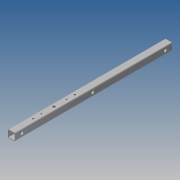
# Autodesk Inventor part: 2f2al
Saved by Autodesk Inventor 2014 SP1 (Build 180222100, 222)
## iProperties
Company: HERA Project
Created: 2013-06-27
Part Number: 2f2al
Material: Steel
Description: Feed backplane support crosspiece
Document SubType Name: Modeling
Designer: David DeBoer
Mass: 345.097 g
Surface Area: 540.887 cm^2
Volume: 43.9614 cm^3
Density: 7.85 g/cm^3
Appearance: Steel
Title: Feed backplane cross
Author: David DeBoer
Autodesk Inventor part; units mm, degrees
ref_plane "YZ Plane" through (0, 0, 0) normal (1, 0, 0) x (0, 1, 0)
ref_plane "XZ Plane" through (0, 0, 0) normal (0, 1, 0) x (-1, 0, 0)
ref_plane "XY Plane" through (0, 0, 0) normal (0, 0, 1) x (1, 0, 0)
sketch "Sketch1" plane through (0, 0, 0) normal (0, 0, 1) x (1, 0, 0)
  line L0 (3.175, 0) -> (22.225, 0)
  line L1 (25.4, 3.175) -> (25.4, 22.225)
  line L2 (22.225, 25.4) -> (3.175, 25.4)
  line L3 (0, 22.225) -> (0, 3.175)
  arc A0 (3.175, 25.4) -> (0, 22.225) centre (3.175, 22.225) ccw
  arc A1 (0, 3.175) -> (3.175, 0) centre (3.175, 3.175) ccw
  arc A2 (22.225, 0) -> (25.4, 3.175) centre (22.225, 3.175) ccw
  arc A3 (25.4, 22.225) -> (22.225, 25.4) centre (22.225, 22.225) ccw
  line L4 (3.175, 23.749) -> (22.225, 23.749)
  arc A4 (23.749, 22.225) -> (22.225, 23.749) centre (22.225, 22.225) ccw
  line L5 (23.749, 22.225) -> (23.749, 3.175)
  arc A5 (22.225, 1.651) -> (23.749, 3.175) centre (22.225, 3.175) ccw
  line L6 (22.225, 1.651) -> (3.175, 1.651)
  arc A6 (1.651, 3.175) -> (3.175, 1.651) centre (3.175, 3.175) ccw
  line L7 (1.651, 3.175) -> (1.651, 22.225)
  arc A7 (3.175, 23.749) -> (1.651, 22.225) centre (3.175, 22.225) ccw
  point P0 (0, 0)
  point P1 (25.4, 0)
  point P2 (0, 25.4)
  dimension "d0" = 25.4
  dimension "d1" = 25.4
  dimension "d2" = 3.175
  dimension "d3" = 1.651
  constraints: 16 end point, 16 point on circle, 8 centre point, 8 tangent, 6 point on line, 4 parallel, 3 equal radius, 2 perpendicular, 1 horizontal, 7 other
  measures "d0" distance of point (0, 0) point (25.4, 0)
  measures "d1" distance of point (0, 25.4) point (0, 0)
  measures "d2" radius of A0
  measures "d3" distance between parallel lines of L4 L2
extrude "Extrusion1" add sketch "Sketch1" along normal blind 299.72
sketch "Sketch2" plane through (3.175, 25.4, 0) normal (0, 1, 0) x (1, 0, 0)
  circle A0 centre (9.525, -149.86) radius 3.175
  line L0 (19.05, -299.72) -> (0, -299.72) projected
  point P0 (-3.175, 0)
  dimension "d6" = 6.35
  dimension "d59" = 149.86
  constraints: 1 centre point
  measures "d6" diameter of A0
  measures "d59" distance from line of L0 A0.centre
hole "Hole1" at (12.7, 25.4, 149.86) direction (0, -1, 0) diameter 9.525 end through all
sketch "Sketch3" plane through (3.175, 25.4, 0) normal (0, 1, 0) x (1, 0, 0)
  circle A0 centre (9.525, -149.86) radius 4.7625 projected
  line L0 (19.05, 0) -> (0, 0) projected
  line L1 (19.05, -299.72) -> (0, -299.72) projected
  line L2 (19.05, 0) -> (19.05, -299.72) projected
  line L3 (9.525, 0) -> (9.525, -299.72) construction
  circle A1 centre (9.525, -76.2) radius 2.6066
  line L4 (9.525, -149.86) -> (19.05, -149.86) construction
  circle A2 centre (9.525, -223.52) radius 2.6066
  point P0 (-3.175, 0)
  dimension "d14" = 76.2
  constraints: 4 end point, 3 midpoint, 2 centre point, 1 point on line, 1 symmetric about line, 1 other
  measures "d14" distance from line of A1.centre L0
hole "Hole2" at (12.7, 25.4, 76.2) at (12.7, 25.4, 223.52) direction (0, -1, 0) diameter 6.35 end through all
sketch "Sketch4" plane through (25.4, 3.175, 0) normal (1, 0, 0) x (0, 0, -1)
  line L0 (0, 19.05) -> (-299.72, 19.05) projected
  line L1 (-299.72, 0) -> (-299.72, 19.05) projected
  line L2 (0, 0) -> (-299.72, 0) projected
  circle A0 centre (-274.32, 9.525) radius 3.2646
  line L3 (-149.86, 19.05) -> (-149.86, 0) construction
  point P0 (0, -3.175)
  dimension "d22" = 25.4
  constraints: 2 end point, 2 midpoint, 1 centre point
  measures "d22" distance from line of A0.centre L1
hole "Hole3" at (25.4, 12.7, 274.32) direction (-1, 0, 0) diameter 9.525 end through all
sketch "Sketch7" plane through (25.4, 3.175, 0) normal (1, 0, 0) x (0, 0, -1)
  line L0 (0, 0) -> (0, 19.05) projected
  circle A0 centre (-25.4, 9.525) radius 3.0513
  point P0 (0, -3.175)
  dimension "d41" = 25.4
  constraints: 1 centre point
  measures "d41" distance from line of A0.centre L0
hole "Hole5" at (25.4, 12.7, 25.4) direction (-1, 0, 0) diameter 9.525 end through all
sketch "Sketch8" plane through (3.175, 25.4, 0) normal (0, 1, 0) x (1, 0, 0)
  circle A0 centre (9.525, -149.86) radius 4.7625 projected
  circle A1 centre (9.525, -194.31) radius 3.5498
  circle A2 centre (9.525, -105.41) radius 3.5498
  point P0 (-3.175, 0)
  dimension "d49" = 44.45
  dimension "d50" = 44.45
  constraints: 2 centre point
  measures "d49" distance of A1.centre A0.centre
  measures "d50" distance of A2.centre A0.centre
hole "Hole6" at (12.7, 25.4, 194.31) at (12.7, 25.4, 105.41) direction (0, -1, 0) diameter 5.1054 depth 25.4 tip angle 118 clearance for "Flat Head Machine Screw (82)" size "#10" standard "Ansi Unified Screw Threads"
sketch "Sketch9" plane through (0, 0, 0) normal (0, 0, -1) x (-1, 0, 0)
  arc A0 (-22.225, 23.749) -> (-23.749, 22.225) centre (-22.225, 22.225) ccw projected
  line L0 (-22.225, 23.749) -> (-3.175, 23.749) projected
  arc A1 (-1.651, 22.225) -> (-3.175, 23.749) centre (-3.175, 22.225) ccw projected
  line L1 (-1.651, 22.225) -> (-1.651, 3.175) projected
  arc A2 (-3.175, 1.651) -> (-1.651, 3.175) centre (-3.175, 3.175) ccw projected
  line L2 (-3.175, 1.651) -> (-22.225, 1.651) projected
  arc A3 (-23.749, 3.175) -> (-22.225, 1.651) centre (-22.225, 3.175) ccw projected
  line L3 (-23.749, 3.175) -> (-23.749, 22.225) projected
  line L4 (0, 22.225) -> (0, 3.175) projected
  arc A4 (0, 22.225) -> (-3.175, 25.4) centre (-3.175, 22.225) ccw projected
  line L5 (-22.225, 25.4) -> (-3.175, 25.4) projected
  arc A5 (-22.225, 25.4) -> (-25.4, 22.225) centre (-22.225, 22.225) ccw projected
  line L6 (-25.4, 3.175) -> (-25.4, 22.225) projected
  arc A6 (-25.4, 3.175) -> (-22.225, 0) centre (-22.225, 3.175) ccw projected
  line L7 (-3.175, 0) -> (-22.225, 0) projected
  arc A7 (-3.175, 0) -> (0, 3.175) centre (-3.175, 3.175) ccw projected
  point P0 (0, 0)
extrude "Extrusion2" add sketch "Sketch9" along normal blind 254
sketch "Sketch10" plane through (25.4, 3.175, 299.72) normal (1, 0, 0) x (0, 0, -1)
  circle A0 centre (530.074, 9.525) radius 4.839
  point P0 (299.72, -3.175)
  constraints: 1 centre point
hole "Hole7" at (25.4, 12.7, -230.354) direction (-1, 0, 0) diameter 9.525 end through all
body "Solid1"
